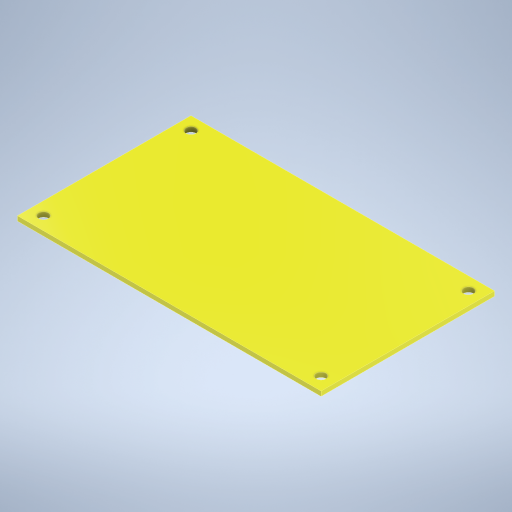
# Autodesk Inventor part: prop_PCB
Saved by Autodesk Inventor 2024.2 (Build 282272000, 272)
## iProperties
Created: 2025-03-01
Part Number: prop_PCB
Material: Všeobecné
Document SubType Name: Modeling
Designer: hepma_axt67em
Density: 1 g/cm^3
Appearance: Žlutá
Author: hepma_axt67em
Autodesk Inventor part; units mm, degrees
ref_plane "YZ Plane" through (0, 0, 0) normal (1, 0, 0) x (0, 1, 0)
ref_plane "XZ Plane" through (0, 0, 0) normal (0, 1, 0) x (-1, 0, 0)
ref_plane "XY Plane" through (0, 0, 0) normal (0, 0, 1) x (1, 0, 0)
sketch "Náčrt1" plane through (0, 0, 0) normal (0, 1, 0) x (-1, 0, 0)
  line L0 (0, -42) -> (0, 42) projected
  line L1 (-73.5, 0) -> (73.5, 0) projected
  line L2 (52.5, 30) -> (-52.5, 30)
  line L3 (-52.5, 30) -> (-52.5, -30)
  line L4 (-52.5, -30) -> (52.5, -30)
  line L5 (52.5, -30) -> (52.5, 30)
  point P0 (0, 0)
  dimension "d0" = 105
  dimension "d1" = 60
  constraints: 8 end point, 2 parallel, 1 horizontal, 1 perpendicular, 2 other
  measures "d0" distance of L4.end L3.end
  measures "d1" distance of L2.end L3.end
extrude "Vysunutí1" add sketch "Náčrt1" along normal blind 1.6
sketch "Náčrt2" plane through (0, 1.6, 0) normal (0, 1, 0) x (1, 0, 0)
  line L0 (0, 42) -> (0, -42) projected
  line L1 (73.5, 0) -> (-73.5, 0) projected
  point P0 (0, 0)
  point P1 (-48, 25.5)
  point P2 (-48, -25.5)
  point P3 (48, -25.5)
  point P4 (48, 25.5)
  dimension "d4" = 96
  dimension "d5" = 51
  dimension "d6" = 51
  dimension "d7" = 96
  dimension "d8" = 48
  dimension "d9" = 25.5
  dimension "d10" = 25.5
  dimension "d11" = 48
  measures "d4" distance of point (48, 25.5) point (-48, 25.5)
  measures "d5" distance of point (48, 25.5) point (48, -25.5)
  measures "d6" distance of point (-48, 25.5) point (-48, -25.5)
  measures "d7" distance of point (48, -25.5) point (-48, -25.5)
  measures "d8" distance from line of L0 point (-48, 25.5)
  measures "d9" distance from line of L1 point (-48, 25.5)
  measures "d10" distance from line of L1 point (48, 25.5)
  measures "d11" distance from line of L0 point (-48, -25.5)
hole "Díra1" at (-48, 1.6, -25.5) at (-48, 1.6, 25.5) at (48, 1.6, 25.5) at (48, 1.6, -25.5) direction (0, -1, 0) diameter 3.4 end through all clearance for "Šroub se zápustnou hlavou ISO 2009/7046" size "M3" standard "ISO"
